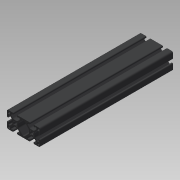
# Autodesk Inventor part: 1530-LS
Saved by Autodesk Inventor 2013 (Build 170138000, 138)
## iProperties
Company: 80/20 Inc.
Created: 2014-04-23
Part Number: 1530-LS
Material: Generic
Document SubType Name: Modeling
Density: 1 g/cm^3
Vendor: 80/20 Inc.
Engineer: Ross Bowman
Designer: Ross Bowman
Catalog Web Link: 8020.net
Material: 6105-T5 Aluminum
Author: Ross Bowman
Keywords: 80/20 , 8020 , T-Slot , Extrusion
Autodesk Inventor part; units mm, degrees
ref_plane "YZ Plane" through (0, 0, 0) normal (1, 0, 0) x (0, 1, 0)
ref_plane "XZ Plane" through (0, 0, 0) normal (0, 1, 0) x (-1, 0, 0)
ref_plane "XY Plane" through (0, 0, 0) normal (0, 0, 1) x (1, 0, 0)
sketch "Sketch1" plane through (0, 0, 0) normal (0, 0, 1) x (1, 0, 0)
  arc A0 (16.4102, 4.2456) -> (14.8044, 2.6398) centre (15.5149, 3.5351) ccw
  line L0 (17.6936, 2.9729) -> (16.4102, 4.2456)
  arc A1 (20.4064, 2.9729) -> (17.6936, 2.9729) centre (19.05, 0) ccw
  line L1 (21.7769, 4.3433) -> (20.4064, 2.9729)
  arc A2 (23.3933, 2.7269) -> (21.7769, 4.3433) centre (22.5851, 3.5351) ccw
  line L2 (22.0229, 1.3564) -> (23.3933, 2.7269)
  arc A3 (22.0229, -1.3564) -> (22.0229, 1.3564) centre (19.05, 0) ccw
  line L3 (23.3933, -2.7269) -> (22.0229, -1.3564)
  arc A4 (21.7769, -4.3433) -> (23.3933, -2.7269) centre (22.5851, -3.5351) ccw
  line L4 (20.4064, -2.9729) -> (21.7769, -4.3433)
  arc A5 (17.6936, -2.9729) -> (20.4064, -2.9729) centre (19.05, 0) ccw
  line L5 (16.3231, -4.3433) -> (17.6936, -2.9729)
  arc A6 (14.7067, -2.7269) -> (16.3231, -4.3433) centre (15.5149, -3.5351) ccw
  line L6 (16.0771, -1.3564) -> (14.7067, -2.7269)
  arc A7 (16.0771, 1.3564) -> (16.0771, -1.3564) centre (19.05, 0) ccw
  line L7 (14.8044, 2.6398) -> (16.0771, 1.3564)
  arc A8 (31.2928, 17.2466) -> (30.9118, 16.8656) centre (31.2928, 16.8656) ccw
  line L8 (33.5026, 17.2466) -> (31.2928, 17.2466)
  arc A9 (36.2966, 14.4526) -> (33.5026, 17.2466) centre (33.5026, 14.4526) ccw
  line L9 (36.2966, 12.2428) -> (36.2966, 14.4526)
  arc A10 (35.9156, 11.8618) -> (36.2966, 12.2428) centre (35.9156, 12.2428) ccw
  line L10 (31.2928, 11.8618) -> (35.9156, 11.8618)
  arc A11 (30.9118, 12.2428) -> (31.2928, 11.8618) centre (31.2928, 12.2428) ccw
  line L11 (30.9118, 16.8656) -> (30.9118, 12.2428)
  arc A12 (36.2966, -12.2428) -> (35.9156, -11.8618) centre (35.9156, -12.2428) ccw
  line L12 (36.2966, -14.4526) -> (36.2966, -12.2428)
  arc A13 (33.5026, -17.2466) -> (36.2966, -14.4526) centre (33.5026, -14.4526) ccw
  line L13 (31.2928, -17.2466) -> (33.5026, -17.2466)
  arc A14 (30.9118, -16.8656) -> (31.2928, -17.2466) centre (31.2928, -16.8656) ccw
  line L14 (30.9118, -12.2428) -> (30.9118, -16.8656)
  arc A15 (31.2928, -11.8618) -> (30.9118, -12.2428) centre (31.2928, -12.2428) ccw
  line L15 (35.9156, -11.8618) -> (31.2928, -11.8618)
  arc A16 (2.0655, 14.8293) -> (-2.0655, 14.8293) centre (0, 12.7638) ccw
  line L16 (10.9278, 5.9669) -> (2.0655, 14.8293)
  arc A17 (12.319, 2.6083) -> (10.9278, 5.9669) centre (7.5692, 2.6083) ccw
  line L17 (12.319, -2.6083) -> (12.319, 2.6083)
  arc A18 (10.9278, -5.9669) -> (12.319, -2.6083) centre (7.5692, -2.6083) ccw
  line L18 (2.0655, -14.8293) -> (10.9278, -5.9669)
  arc A19 (-2.0655, -14.8293) -> (2.0655, -14.8293) centre (0, -12.7638) ccw
  line L19 (-10.9278, -5.9669) -> (-2.0655, -14.8293)
  arc A20 (-12.319, -2.6083) -> (-10.9278, -5.9669) centre (-7.5692, -2.6083) ccw
  line L20 (-12.319, 2.6083) -> (-12.319, -2.6083)
  arc A21 (-10.9278, 5.9669) -> (-12.319, 2.6083) centre (-7.5692, 2.6083) ccw
  line L21 (-2.0655, 14.8293) -> (-10.9278, 5.9669)
  arc A22 (-14.8044, 2.6398) -> (-16.4102, 4.2456) centre (-15.5149, 3.5351) ccw
  line L22 (-16.0771, 1.3564) -> (-14.8044, 2.6398)
  arc A23 (-16.0771, -1.3564) -> (-16.0771, 1.3564) centre (-19.05, 0) ccw
  line L23 (-14.7067, -2.7269) -> (-16.0771, -1.3564)
  arc A24 (-16.3231, -4.3433) -> (-14.7067, -2.7269) centre (-15.5149, -3.5351) ccw
  line L24 (-17.6936, -2.9729) -> (-16.3231, -4.3433)
  arc A25 (-20.4064, -2.9729) -> (-17.6936, -2.9729) centre (-19.05, 0) ccw
  line L25 (-21.7769, -4.3433) -> (-20.4064, -2.9729)
  arc A26 (-23.3933, -2.7269) -> (-21.7769, -4.3433) centre (-22.5851, -3.5351) ccw
  line L26 (-22.0229, -1.3564) -> (-23.3933, -2.7269)
  arc A27 (-22.0229, 1.3564) -> (-22.0229, -1.3564) centre (-19.05, 0) ccw
  line L27 (-23.3933, 2.7269) -> (-22.0229, 1.3564)
  arc A28 (-21.7769, 4.3433) -> (-23.3933, 2.7269) centre (-22.5851, 3.5351) ccw
  line L28 (-20.4064, 2.9729) -> (-21.7769, 4.3433)
  arc A29 (-17.6936, 2.9729) -> (-20.4064, 2.9729) centre (-19.05, 0) ccw
  line L29 (-16.4102, 4.2456) -> (-17.6936, 2.9729)
  arc A30 (-30.9118, 16.8656) -> (-31.2928, 17.2466) centre (-31.2928, 16.8656) ccw
  line L30 (-30.9118, 12.2428) -> (-30.9118, 16.8656)
  arc A31 (-31.2928, 11.8618) -> (-30.9118, 12.2428) centre (-31.2928, 12.2428) ccw
  line L31 (-35.9156, 11.8618) -> (-31.2928, 11.8618)
  arc A32 (-36.2966, 12.2428) -> (-35.9156, 11.8618) centre (-35.9156, 12.2428) ccw
  line L32 (-36.2966, 14.4526) -> (-36.2966, 12.2428)
  arc A33 (-33.5026, 17.2466) -> (-36.2966, 14.4526) centre (-33.5026, 14.4526) ccw
  line L33 (-31.2928, 17.2466) -> (-33.5026, 17.2466)
  arc A34 (-35.9156, -11.8618) -> (-36.2966, -12.2428) centre (-35.9156, -12.2428) ccw
  line L34 (-31.2928, -11.8618) -> (-35.9156, -11.8618)
  arc A35 (-30.9118, -12.2428) -> (-31.2928, -11.8618) centre (-31.2928, -12.2428) ccw
  line L35 (-30.9118, -16.8656) -> (-30.9118, -12.2428)
  arc A36 (-31.2928, -17.2466) -> (-30.9118, -16.8656) centre (-31.2928, -16.8656) ccw
  line L36 (-33.5026, -17.2466) -> (-31.2928, -17.2466)
  arc A37 (-36.2966, -14.4526) -> (-33.5026, -17.2466) centre (-33.5026, -14.4526) ccw
  line L37 (-36.2966, -12.2428) -> (-36.2966, -14.4526)
  arc A38 (34.8742, 9.013) -> (33.6042, 10.287) centre (33.6042, 9.017) ccw
  line L38 (34.8742, 9.013) -> (34.8742, 7.239)
  arc A39 (34.4932, 6.858) -> (34.8742, 7.239) centre (34.4932, 7.239) ccw
  line L39 (34.4932, 6.858) -> (34.417, 6.858)
  arc A40 (34.417, 6.858) -> (34.036, 6.477) centre (34.417, 6.477) ccw
  line L40 (34.036, 6.477) -> (34.036, 5.6388)
  arc A41 (34.036, 5.6388) -> (35.6108, 4.064) centre (35.6108, 5.6388) ccw
  line L41 (35.6108, 4.064) -> (36.5252, 4.064)
  arc A42 (36.5252, 4.064) -> (38.1, 5.6388) centre (36.5252, 5.6388) ccw
  line L42 (38.1, 5.6388) -> (38.1, 15.875)
  arc A43 (38.1, 15.875) -> (34.925, 19.05) centre (34.925, 15.875) ccw
  line L43 (34.925, 19.05) -> (24.6888, 19.05)
  arc A44 (24.6888, 19.05) -> (23.114, 17.4752) centre (24.6888, 17.4752) ccw
  line L44 (23.114, 17.4752) -> (23.114, 16.5608)
  arc A45 (23.114, 16.5608) -> (24.6888, 14.986) centre (24.6888, 16.5608) ccw
  line L45 (24.6888, 14.986) -> (25.527, 14.986)
  arc A46 (25.527, 14.986) -> (25.908, 15.367) centre (25.527, 15.367) ccw
  line L46 (25.908, 15.367) -> (25.908, 15.4432)
  arc A47 (26.289, 15.8242) -> (25.908, 15.4432) centre (26.289, 15.4432) ccw
  line L47 (26.289, 15.8242) -> (28.063, 15.8242)
  arc A48 (29.337, 14.5542) -> (28.063, 15.8242) centre (28.067, 14.5542) ccw
  line L48 (29.337, 14.5542) -> (29.337, 12.9683)
  arc A49 (28.965, 12.0703) -> (29.337, 12.9683) centre (28.067, 12.9683) ccw
  line L49 (28.965, 12.0703) -> (25.0169, 8.1222)
  arc A50 (21.6583, 6.731) -> (25.0169, 8.1222) centre (21.6583, 11.4808) ccw
  line L50 (21.6583, 6.731) -> (16.4417, 6.731)
  arc A51 (13.0831, 8.1222) -> (16.4417, 6.731) centre (16.4417, 11.4808) ccw
  line L51 (13.0831, 8.1222) -> (9.135, 12.0703)
  arc A52 (8.763, 12.9683) -> (9.135, 12.0703) centre (10.033, 12.9683) ccw
  line L52 (8.763, 12.9683) -> (8.763, 14.5542)
  arc A53 (10.033, 15.8242) -> (8.763, 14.5542) centre (10.033, 14.5542) ccw
  line L53 (10.033, 15.8242) -> (11.811, 15.8242)
  arc A54 (12.192, 15.4432) -> (11.811, 15.8242) centre (11.811, 15.4432) ccw
  line L54 (12.192, 15.4432) -> (12.192, 15.367)
  arc A55 (12.192, 15.367) -> (12.573, 14.986) centre (12.573, 15.367) ccw
  line L55 (12.573, 14.986) -> (13.4112, 14.986)
  arc A56 (13.4112, 14.986) -> (14.986, 16.5608) centre (13.4112, 16.5608) ccw
  line L56 (14.986, 16.5608) -> (14.986, 17.4752)
  arc A57 (14.986, 17.4752) -> (13.4112, 19.05) centre (13.4112, 17.4752) ccw
  line L57 (13.4112, 19.05) -> (-13.4112, 19.05)
  arc A58 (-13.4112, 19.05) -> (-14.986, 17.4752) centre (-13.4112, 17.4752) ccw
  line L58 (-14.986, 17.4752) -> (-14.986, 16.5608)
  arc A59 (-14.986, 16.5608) -> (-13.4112, 14.986) centre (-13.4112, 16.5608) ccw
  line L59 (-13.4112, 14.986) -> (-12.573, 14.986)
  arc A60 (-12.573, 14.986) -> (-12.192, 15.367) centre (-12.573, 15.367) ccw
  line L60 (-12.192, 15.367) -> (-12.192, 15.4432)
  arc A61 (-11.811, 15.8242) -> (-12.192, 15.4432) centre (-11.811, 15.4432) ccw
  line L61 (-11.811, 15.8242) -> (-10.037, 15.8242)
  arc A62 (-8.763, 14.5542) -> (-10.037, 15.8242) centre (-10.033, 14.5542) ccw
  line L62 (-8.763, 14.5542) -> (-8.763, 12.9683)
  arc A63 (-9.135, 12.0703) -> (-8.763, 12.9683) centre (-10.033, 12.9683) ccw
  line L63 (-9.135, 12.0703) -> (-13.0831, 8.1222)
  arc A64 (-16.4417, 6.731) -> (-13.0831, 8.1222) centre (-16.4417, 11.4808) ccw
  line L64 (-16.4417, 6.731) -> (-21.6583, 6.731)
  arc A65 (-25.0169, 8.1222) -> (-21.6583, 6.731) centre (-21.6583, 11.4808) ccw
  line L65 (-25.0169, 8.1222) -> (-28.965, 12.0703)
  arc A66 (-29.337, 12.9683) -> (-28.965, 12.0703) centre (-28.067, 12.9683) ccw
  line L66 (-29.337, 12.9683) -> (-29.337, 14.5542)
  arc A67 (-28.067, 15.8242) -> (-29.337, 14.5542) centre (-28.067, 14.5542) ccw
  line L67 (-28.067, 15.8242) -> (-26.289, 15.8242)
  arc A68 (-25.908, 15.4432) -> (-26.289, 15.8242) centre (-26.289, 15.4432) ccw
  line L68 (-25.908, 15.4432) -> (-25.908, 15.367)
  arc A69 (-25.908, 15.367) -> (-25.527, 14.986) centre (-25.527, 15.367) ccw
  line L69 (-25.527, 14.986) -> (-24.6888, 14.986)
  arc A70 (-24.6888, 14.986) -> (-23.114, 16.5608) centre (-24.6888, 16.5608) ccw
  line L70 (-23.114, 16.5608) -> (-23.114, 17.4752)
  arc A71 (-23.114, 17.4752) -> (-24.6888, 19.05) centre (-24.6888, 17.4752) ccw
  line L71 (-24.6888, 19.05) -> (-34.925, 19.05)
  arc A72 (-34.925, 19.05) -> (-38.1, 15.875) centre (-34.925, 15.875) ccw
  line L72 (-38.1, 15.875) -> (-38.1, 5.6388)
  arc A73 (-38.1, 5.6388) -> (-36.5252, 4.064) centre (-36.5252, 5.6388) ccw
  line L73 (-36.5252, 4.064) -> (-35.6108, 4.064)
  arc A74 (-35.6108, 4.064) -> (-34.036, 5.6388) centre (-35.6108, 5.6388) ccw
  line L74 (-34.036, 5.6388) -> (-34.036, 6.477)
  arc A75 (-34.036, 6.477) -> (-34.417, 6.858) centre (-34.417, 6.477) ccw
  line L75 (-34.417, 6.858) -> (-34.4932, 6.858)
  arc A76 (-34.8742, 7.239) -> (-34.4932, 6.858) centre (-34.4932, 7.239) ccw
  line L76 (-34.8742, 7.239) -> (-34.8742, 9.013)
  arc A77 (-33.6042, 10.287) -> (-34.8742, 9.013) centre (-33.6042, 9.017) ccw
  line L77 (-33.6042, 10.287) -> (-32.0183, 10.287)
  arc A78 (-31.1203, 9.915) -> (-32.0183, 10.287) centre (-32.0183, 9.017) ccw
  line L78 (-31.1203, 9.915) -> (-27.1722, 5.9669)
  arc A79 (-25.781, 2.6083) -> (-27.1722, 5.9669) centre (-30.5308, 2.6083) ccw
  line L79 (-25.781, 2.6083) -> (-25.781, -2.6083)
  arc A80 (-27.1722, -5.9669) -> (-25.781, -2.6083) centre (-30.5308, -2.6083) ccw
  line L80 (-27.1722, -5.9669) -> (-31.1203, -9.915)
  arc A81 (-32.0183, -10.287) -> (-31.1203, -9.915) centre (-32.0183, -9.017) ccw
  line L81 (-32.0183, -10.287) -> (-33.6042, -10.287)
  arc A82 (-34.8742, -9.017) -> (-33.6042, -10.287) centre (-33.6042, -9.017) ccw
  line L82 (-34.8742, -9.017) -> (-34.8742, -7.239)
  arc A83 (-34.4932, -6.858) -> (-34.8742, -7.239) centre (-34.4932, -7.239) ccw
  line L83 (-34.4932, -6.858) -> (-34.417, -6.858)
  arc A84 (-34.417, -6.858) -> (-34.036, -6.477) centre (-34.417, -6.477) ccw
  line L84 (-34.036, -6.477) -> (-34.036, -5.6388)
  arc A85 (-34.036, -5.6388) -> (-35.6108, -4.064) centre (-35.6108, -5.6388) ccw
  line L85 (-35.6108, -4.064) -> (-36.5252, -4.064)
  arc A86 (-36.5252, -4.064) -> (-38.1, -5.6388) centre (-36.5252, -5.6388) ccw
  line L86 (-38.1, -5.6388) -> (-38.1, -15.875)
  arc A87 (-38.1, -15.875) -> (-34.925, -19.05) centre (-34.925, -15.875) ccw
  line L87 (-34.925, -19.05) -> (-24.6888, -19.05)
  arc A88 (-24.6888, -19.05) -> (-23.114, -17.4752) centre (-24.6888, -17.4752) ccw
  line L88 (-23.114, -17.4752) -> (-23.114, -16.5608)
  arc A89 (-23.114, -16.5608) -> (-24.6888, -14.986) centre (-24.6888, -16.5608) ccw
  line L89 (-24.6888, -14.986) -> (-25.527, -14.986)
  arc A90 (-25.527, -14.986) -> (-25.908, -15.367) centre (-25.527, -15.367) ccw
  line L90 (-25.908, -15.367) -> (-25.908, -15.4432)
  arc A91 (-26.289, -15.8242) -> (-25.908, -15.4432) centre (-26.289, -15.4432) ccw
  line L91 (-26.289, -15.8242) -> (-28.063, -15.8242)
  arc A92 (-29.337, -14.5542) -> (-28.063, -15.8242) centre (-28.067, -14.5542) ccw
  line L92 (-29.337, -14.5542) -> (-29.337, -12.9683)
  arc A93 (-28.965, -12.0703) -> (-29.337, -12.9683) centre (-28.067, -12.9683) ccw
  line L93 (-28.965, -12.0703) -> (-25.0169, -8.1222)
  arc A94 (-21.6583, -6.731) -> (-25.0169, -8.1222) centre (-21.6583, -11.4808) ccw
  line L94 (-21.6583, -6.731) -> (-16.4417, -6.731)
  arc A95 (-13.0831, -8.1222) -> (-16.4417, -6.731) centre (-16.4417, -11.4808) ccw
  line L95 (-13.0831, -8.1222) -> (-9.135, -12.0703)
  arc A96 (-8.763, -12.9683) -> (-9.135, -12.0703) centre (-10.033, -12.9683) ccw
  line L96 (-8.763, -12.9683) -> (-8.763, -14.5542)
  arc A97 (-10.033, -15.8242) -> (-8.763, -14.5542) centre (-10.033, -14.5542) ccw
  line L97 (-10.033, -15.8242) -> (-11.811, -15.8242)
  arc A98 (-12.192, -15.4432) -> (-11.811, -15.8242) centre (-11.811, -15.4432) ccw
  line L98 (-12.192, -15.4432) -> (-12.192, -15.367)
  arc A99 (-12.192, -15.367) -> (-12.573, -14.986) centre (-12.573, -15.367) ccw
  line L99 (-12.573, -14.986) -> (-13.4112, -14.986)
  arc A100 (-13.4112, -14.986) -> (-14.986, -16.5608) centre (-13.4112, -16.5608) ccw
  line L100 (-14.986, -16.5608) -> (-14.986, -17.4752)
  arc A101 (-14.986, -17.4752) -> (-13.4112, -19.05) centre (-13.4112, -17.4752) ccw
  line L101 (-13.4112, -19.05) -> (13.4112, -19.05)
  arc A102 (13.4112, -19.05) -> (14.986, -17.4752) centre (13.4112, -17.4752) ccw
  line L102 (14.986, -17.4752) -> (14.986, -16.5608)
  arc A103 (14.986, -16.5608) -> (13.4112, -14.986) centre (13.4112, -16.5608) ccw
  line L103 (13.4112, -14.986) -> (12.573, -14.986)
  arc A104 (12.573, -14.986) -> (12.192, -15.367) centre (12.573, -15.367) ccw
  line L104 (12.192, -15.367) -> (12.192, -15.4432)
  arc A105 (11.811, -15.8242) -> (12.192, -15.4432) centre (11.811, -15.4432) ccw
  line L105 (11.811, -15.8242) -> (10.037, -15.8242)
  arc A106 (8.763, -14.5542) -> (10.037, -15.8242) centre (10.033, -14.5542) ccw
  line L106 (8.763, -14.5542) -> (8.763, -12.9683)
  arc A107 (9.135, -12.0703) -> (8.763, -12.9683) centre (10.033, -12.9683) ccw
  line L107 (9.135, -12.0703) -> (13.0831, -8.1222)
  arc A108 (16.4417, -6.731) -> (13.0831, -8.1222) centre (16.4417, -11.4808) ccw
  line L108 (16.4417, -6.731) -> (21.6583, -6.731)
  arc A109 (25.0169, -8.1222) -> (21.6583, -6.731) centre (21.6583, -11.4808) ccw
  line L109 (25.0169, -8.1222) -> (28.965, -12.0703)
  arc A110 (29.337, -12.9683) -> (28.965, -12.0703) centre (28.067, -12.9683) ccw
  line L110 (29.337, -12.9683) -> (29.337, -14.5542)
  arc A111 (28.067, -15.8242) -> (29.337, -14.5542) centre (28.067, -14.5542) ccw
  line L111 (28.067, -15.8242) -> (26.289, -15.8242)
  arc A112 (25.908, -15.4432) -> (26.289, -15.8242) centre (26.289, -15.4432) ccw
  line L112 (25.908, -15.4432) -> (25.908, -15.367)
  arc A113 (25.908, -15.367) -> (25.527, -14.986) centre (25.527, -15.367) ccw
  line L113 (25.527, -14.986) -> (24.6888, -14.986)
  arc A114 (24.6888, -14.986) -> (23.114, -16.5608) centre (24.6888, -16.5608) ccw
  line L114 (23.114, -16.5608) -> (23.114, -17.4752)
  arc A115 (23.114, -17.4752) -> (24.6888, -19.05) centre (24.6888, -17.4752) ccw
  line L115 (24.6888, -19.05) -> (34.925, -19.05)
  arc A116 (34.925, -19.05) -> (38.1, -15.875) centre (34.925, -15.875) ccw
  line L116 (38.1, -15.875) -> (38.1, -5.6388)
  arc A117 (38.1, -5.6388) -> (36.5252, -4.064) centre (36.5252, -5.6388) ccw
  line L117 (36.5252, -4.064) -> (35.6108, -4.064)
  arc A118 (35.6108, -4.064) -> (34.036, -5.6388) centre (35.6108, -5.6388) ccw
  line L118 (34.036, -5.6388) -> (34.036, -6.477)
  arc A119 (34.036, -6.477) -> (34.417, -6.858) centre (34.417, -6.477) ccw
  line L119 (34.417, -6.858) -> (34.4932, -6.858)
  arc A120 (34.8742, -7.239) -> (34.4932, -6.858) centre (34.4932, -7.239) ccw
  line L120 (34.8742, -7.239) -> (34.8742, -9.013)
  arc A121 (33.6042, -10.287) -> (34.8742, -9.013) centre (33.6042, -9.017) ccw
  line L121 (33.6042, -10.287) -> (32.0183, -10.287)
  arc A122 (31.1203, -9.915) -> (32.0183, -10.287) centre (32.0183, -9.017) ccw
  line L122 (31.1203, -9.915) -> (27.1722, -5.9669)
  arc A123 (25.781, -2.6083) -> (27.1722, -5.9669) centre (30.5308, -2.6083) ccw
  line L123 (25.781, -2.6083) -> (25.781, 2.6083)
  arc A124 (27.1722, 5.9669) -> (25.781, 2.6083) centre (30.5308, 2.6083) ccw
  line L124 (27.1722, 5.9669) -> (31.1203, 9.915)
  arc A125 (32.0183, 10.287) -> (31.1203, 9.915) centre (32.0183, 9.017) ccw
  line L125 (32.0183, 10.287) -> (33.6042, 10.287)
  point P0 (0, 0)
  constraints: 252 end point, 252 point on circle, 126 centre point
extrude "Extrusion1" add sketch "Sketch1" against normal blind 304.8
body "Solid1"
